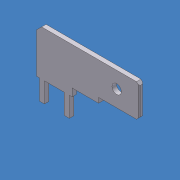
# Autodesk Inventor part: Spike Male Terminal
Saved by Autodesk Inventor 2012 (Build 160160000, 160)
## iProperties
Shininess: 64.0
Length Units: 11269
Angle Units: 11279
Time Units: 11290
Mass Units: 11283
Length Display Precision: 3
Angle Display Precision: 2
Compacted: True
Part Number: Spike Male Terminal
Document SubType Name: Modeling
Created: 2006-01-06
Material: Steel, Mild
Designer: Owner
Density: 1 g/cm^3
Density: 0.0
Volumn: 0.0
Area: 0.0
PropertySet Name: Model Information
Control State: 0
Master: False
Checked Out: False
Author: Owner
Autodesk Inventor part; units mm, degrees
ref_plane "YZ Plane" through (0, 0, 0) normal (1, 0, 0) x (0, 1, 0)
ref_plane "XZ Plane" through (0, 0, 0) normal (0, 1, 0) x (-1, 0, 0)
ref_plane "XY Plane" through (0, 0, 0) normal (0, 0, 1) x (1, 0, 0)
sketch "Sketch1" plane through (0, 0, 0) normal (0, 0, 1) x (1, 0, 0)
  line L0 (0, -8.9) -> (0, 0)
  line L1 (0, 0) -> (20.15, 0)
  line L2 (20.15, 0) -> (20.15, -6.4)
  line L3 (20.15, -6.4) -> (12.2, -6.4)
  line L4 (12.2, -6.4) -> (12.2, -7.4)
  line L5 (12.2, -7.4) -> (7, -7.4)
  line L6 (7, -7.4) -> (7, -8.9)
  line L7 (7, -8.9) -> (6.45, -8.9)
  line L8 (6.45, -8.9) -> (6.45, -12.85)
  line L9 (6.45, -12.85) -> (5.45, -12.85)
  line L10 (5.45, -12.85) -> (5.45, -8.9)
  line L11 (5.45, -8.9) -> (1.55, -8.9)
  line L12 (1.55, -8.9) -> (1.55, -12.85)
  line L13 (1.55, -12.85) -> (0.55, -12.85)
  line L14 (0.55, -12.85) -> (0.55, -8.9)
  line L15 (0.55, -8.9) -> (0, -8.9)
  dimension "d0" = 20.15
  dimension "d1" = 1
  dimension "d2" = 7
  dimension "d3" = 3.9
  dimension "d4" = 1.5
  dimension "d5" = 1
  dimension "d6" = 7.4
  dimension "d7" = 12.2
  dimension "d9" = 12.85
  constraints: 32 end point, 8 horizontal, 8 vertical, 5 equal length, 1 other
  measures "d0" distance of L0.end L1.end
  measures "d1" distance of L12.end L13.end
  measures "d2" distance between parallel lines of L6 L0
  measures "d3" distance of L10.end L11.end
  measures "d4" distance of L5.end L6.end
  measures "d5" distance of L3.end L4.end
  measures "d6" distance between parallel lines of L1 L5
  measures "d7" distance between parallel lines of L0 L4
  measures "d9" distance between parallel lines of L13 L1
extrude "Extrusion1" add sketch "Sketch1" along normal blind 0.87
sketch "Sketch2" plane through (0, 0, 0.87) normal (0, 0, 1) x (1, 0, 0)
  line L0 (0, 0) -> (20.15, 0) projected
  line L1 (20.15, -6.4) -> (12.2, -6.4) projected
  line L2 (20.15, 0) -> (20.15, -6.4) projected
  line L3 (15.75, -3.2) -> (15.75, 0) construction
  line L4 (15.75, -3.2) -> (15.75, -6.4) construction
  dimension "d13" = 4.4
  constraints: 4 end point, 2 point on line, 2 vertical, 1 collinear
  measures "d13" distance from line of L2 L3.start
hole "Hole1" at (15.75, -3.2, 0.87) direction (0, 0, -1) diameter 1.85 end through all
chamfer "Chamfer1" distance 0.5 angle 45 2 edges at (20.15, -6.4, 0.435) (20.15, 0, 0.435)
chamfer "Chamfer2" distance 0.2 angle 45 2 edges at (20.15, -3.2, 0.87) (20.15, -3.2, 0)
chamfer "Chamfer3" distance 1 angle 45 1 edges at (0, 0, 0.435)
body "Solid1"
